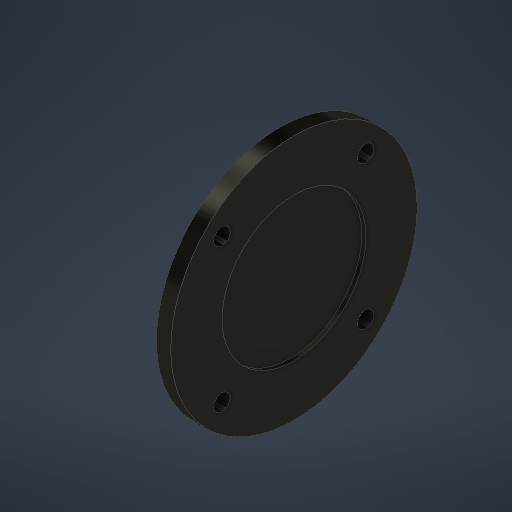
# Autodesk Inventor part: Diff_CV_Output_V1
Saved by Autodesk Inventor 2026.1 (Build 301233000, 233)
## iProperties
Created: 2026-08-05
Part Number: Diff_CV_Output_V1
Material: Generic
Document SubType Name: Modeling
Designer: share
Density: 1 g/cm^3
Appearance: Default
Author: share
Autodesk Inventor part; units mm, degrees
ref_plane "YZ Plane" through (0, 0, 0) normal (1, 0, 0) x (0, 1, 0)
ref_plane "XZ Plane" through (0, 0, 0) normal (0, 1, 0) x (-1, 0, 0)
ref_plane "XY Plane" through (0, 0, 0) normal (0, 0, 1) x (1, 0, 0)
sketch "Sketch1" plane through (0, 0, 0) normal (1, 0, 0) x (0, 1, 0)
  circle A0 centre (0, 0) radius 60
  line L0 (0, 84) -> (0, -84) construction
  line L1 (-84, 0) -> (84, 0) construction
  dimension "d0" = 120
  constraints: 1 centre point, 1 coincident
  measures "d0" diameter of A0
extrude "Flange" add sketch "Sketch1" against normal blind 7
sketch "Sketch2" plane through (0, 0, 0) normal (1, 0, 0) x (0, 0, -1)
  line L0 (-84, 0) -> (84, 0) construction
  line L1 (0, -84) -> (0, 84) construction
  point P0 (0, 0)
  point P1 (-35, 35)
  point P2 (35, 35)
  point P3 (35, -35)
  point P4 (-35, -35)
  dimension "d5" = 70
  dimension "d6" = 70
  constraints: 3 symmetric about line
  measures "d5" distance of point (35, 35) point (-35, 35)
  measures "d6" distance of point (-35, -35) point (-35, 35)
hole "Bolt Holes" at (0, 35, 35) at (0, 35, -35) at (0, -35, -35) at (0, -35, 35) direction (-1, 0, 0) diameter 8 end through all
sketch "Sketch3" plane through (-7, 0, 0) normal (-1, 0, 0) x (0, 0, 1)
  circle A0 centre (0, 0) radius 10
  dimension "d14" = 20
  constraints: 1 centre point, 1 coincident
  measures "d14" diameter of A0
extrude "CV Input" add sketch "Sketch3" along normal blind 30
sketch "Sketch4" plane through (0, 0, 0) normal (1, 0, 0) x (0, 0, -1)
  circle A0 centre (0, 0) radius 35
  dimension "d20" = 70
  constraints: 1 centre point, 1 coincident
  measures "d20" diameter of A0
extrude "Extrusion3" cut sketch "Sketch4" against normal blind 2
body "Solid1"
